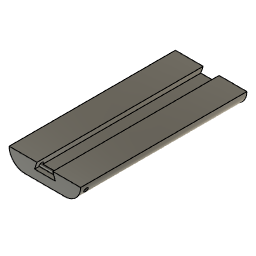
Base Slip Cover v1 (Autodesk Fusion 360 design; units mm, degrees)
Autodesk Fusion 360 part; units mm, degrees
sketch "Sketch1" plane through (0, 0, 0) normal (0, 1, 0) x (1, 0, 0)
  line L0 (0, 0) -> (37, 0)
  line L1 (37, 0) -> (37, -8.15)
  line L2 (37, -8.15) -> (0, -8.15)
  line L3 (0, -8.15) -> (0, 0)
  line L4 (37, -8.15) -> (28.85, -8.15)
  line L5 (28.85, -8.15) -> (28.85, 0)
  line L6 (28.85, 0) -> (37, 0)
  line L7 (37, 0) -> (37, -8.15)
  arc A0 (37, -8.15) -> (28.85, 0) centre (28.85, -8.15) ccw
  line L8 (0, -8.15) -> (8.15, -8.15)
  line L9 (8.15, -8.15) -> (8.15, 0)
  line L10 (8.15, 0) -> (0, 0)
  line L11 (0, 0) -> (0, -8.15)
  arc A1 (8.15, 0) -> (0, -8.15) centre (8.15, -8.15) ccw
  dimension "d1" = 37
  dimension "d2" = 8.15
  dimension "d3" = 8.15
  dimension "d4" = 8.15
  dimension "d5" = 8.15
  dimension "d6" = 8.15
  constraint horizontal L0
  constraint vertical L1
  constraint horizontal L2
  constraint vertical L3
  constraint coincident L0.start L3.end
  constraint horizontal L4
  constraint vertical L5
  constraint horizontal L6
  constraint vertical L7
  constraint tangent L7 A0
  constraint horizontal L8
  constraint vertical L9
  constraint horizontal L10
  constraint vertical L11
  constraint tangent L0 A1
  measures "d1" distance of L0.start L0.end
  measures "d2" distance of L0.start L2.end
  measures "d3" distance of L1.end L4.end
  measures "d4" distance of L1.end L0.end
  measures "d5" distance of L2.end L0.start
  measures "d6" distance of L2.end L8.end
extrude "Extrude1" add sketch "Sketch1" along normal blind 86 contours L0 L2 L5 L9 | L2 L8 L9 A1 | L2 L4 L5 A0
sketch "Sketch2" plane through (0, 0, 0) normal (0, -1, 0) x (1, 0, 0)
  arc A0 (28.85, 0) -> (37, 8.15) centre (28.85, 8.15) ccw
  line L0 (37, 8.15) -> (0, 8.15)
  arc A1 (0, 8.15) -> (8.15, 0) centre (8.15, 8.15) ccw
  line L1 (8.15, 0) -> (28.85, 0)
  line L2 (18.5, 8.15) -> (18.5, 0)
  line L3 (13.125, 4.48) -> (23.875, 4.48)
  line L4 (14.4, 8.15) -> (22.6, 8.15)
  line L5 (14.4, 8.15) -> (13.125, 4.48)
  line L6 (22.6, 8.15) -> (23.875, 4.48)
  dimension "d9" = 10.75
  dimension "d10" = 3.67
  dimension "d11" = 8.2
  constraint midpoint L0 L2.start
  constraint midpoint L1 L2.end
  constraint perpendicular L2 L3
  constraint perpendicular L2 L4
  constraint midpoint L0 L4
  measures "d9" distance of L3.start L3.end
  measures "d10" distance of L0 L3
  measures "d11" distance of L4.start L4.end
extrude "Extrude2" cut sketch "Sketch2" against normal blind 115 contours L0 L2 L3 L4 L6 | L0 L2 L3 L4 L5
sketch "Sketch3" plane through (0, 0, 0) normal (1, 0, 0) x (0, 1, 0)
  circle A0 centre (3.3767, 5.025) radius 1.125
  line L0 (-5, 8) -> (-5, 0)
  line L1 (-3.6483, 8.15) -> (5, 8.15)
  line L2 (5, 8.15) -> (5, -1.85)
  line L3 (5, -1.85) -> (-3.6483, -1.85)
  line L4 (-3.6483, -1.85) -> (-3.6483, 8.15)
  line L5 (0, 8.15) -> (86, 8.15)
  dimension "d14" = 2.25
  dimension "d16" = 5.9
  dimension "d17" = 2
  constraint vertical L0
  constraint horizontal L1
  constraint vertical L2
  constraint horizontal L3
  constraint vertical L4
  constraint collinear L1 L5
  measures "d14" diameter of A0
  measures "d16" distance of A0 L4
  measures "d17" distance of A0 L1
extrude "Extrude3" cut sketch "Sketch3" along normal blind 48 contours A0
